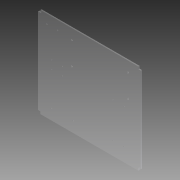
# Autodesk Inventor part: base plate
Saved by Autodesk Inventor 2012 (Build 160160000, 160)
## iProperties
Created: 2012-03-15
Part Number: base plate
Material: Polycarbonate, Clear
Document SubType Name: Modeling
Designer: Ed
Mass: 1928.1 g
Surface Area: 5188.7 cm^2
Volume: 1606.75 cm^3
Density: 1.2 g/cm^3
Author: Ed
Autodesk Inventor part; units mm, degrees
ref_plane "YZ Plane" through (0, 0, 0) normal (1, 0, 0) x (0, 1, 0)
ref_plane "XZ Plane" through (0, 0, 0) normal (0, 1, 0) x (-1, 0, 0)
ref_plane "XY Plane" through (0, 0, 0) normal (0, 0, 1) x (1, 0, 0)
sketch "Sketch1" plane through (0, 0, 0) normal (0, 0, 1) x (1, 0, 0)
  line L0 (0, 0) -> (546.1, 0)
  line L1 (546.1, 0) -> (546.1, 479.425)
  line L2 (546.1, 479.425) -> (0, 479.425)
  line L3 (0, 479.425) -> (0, 0)
  line L4 (0, 0) -> (12.7, 0)
  line L5 (12.7, 0) -> (12.7, 12.7)
  line L6 (12.7, 12.7) -> (0, 12.7)
  line L7 (0, 12.7) -> (0, 0)
  line L8 (0, 479.425) -> (12.7, 479.425)
  line L9 (12.7, 479.425) -> (12.7, 466.725)
  line L10 (12.7, 466.725) -> (0, 466.725)
  line L11 (0, 466.725) -> (0, 479.425)
  line L12 (546.1, 479.425) -> (533.4, 479.425)
  line L13 (533.4, 479.425) -> (533.4, 466.725)
  line L14 (533.4, 466.725) -> (546.1, 466.725)
  line L15 (546.1, 466.725) -> (546.1, 479.425)
  line L16 (546.1, 0) -> (533.4, 0)
  line L17 (533.4, 0) -> (533.4, 12.7)
  line L18 (533.4, 12.7) -> (546.1, 12.7)
  line L19 (546.1, 12.7) -> (546.1, 0)
  dimension "d0" = 479.425
  dimension "d1" = 546.1
  dimension "d2" = 12.7
  constraints: 40 end point, 10 parallel, 7 equal length, 5 horizontal, 5 perpendicular
  measures "d0" distance of L2.end L0.start
  measures "d1" distance of L0.start L0.end
  measures "d2" distance of L8.end L9.end
extrude "Lexan Plate" add sketch "Sketch1" along normal blind 6.35 contours L5 L6 L3 L10 L9 L2 L13 L14 L1 L18 L17 L0
sketch "Sketch2" plane through (0, 0, 6.35) normal (0, 0, 1) x (1, 0, 0)
  line L0 (12.7, 479.425) -> (533.4, 479.425) projected
  line L1 (546.1, 466.725) -> (546.1, 12.7) projected
  line L2 (476.25, 301.625) -> (177.8, 301.625)
  line L3 (177.8, 301.625) -> (177.8, 422.275)
  line L4 (177.8, 422.275) -> (476.25, 422.275)
  line L5 (476.25, 422.275) -> (476.25, 301.625)
  point P0 (0, 0)
  dimension "d7" = 69.85
  dimension "d8" = 57.15
  dimension "d9" = 120.65
  dimension "d10" = 298.45
  constraints: 8 end point, 4 coincident, 2 parallel, 1 horizontal, 1 perpendicular
  measures "d7" distance between parallel lines of L1 L5
  measures "d8" distance between parallel lines of L4 L0
  measures "d9" distance of L4.end L2.start
  measures "d10" distance of L3.end L4.end
hole "Inverter Mounting Holes" at (177.8, 422.275, 6.35) at (177.8, 301.625, 6.35) at (476.25, 301.625, 6.35) at (476.25, 422.275, 6.35) direction (0, 0, -1) diameter 6.7564 end through all clearance for "Flat Head Machine Screw (82)" size "1/4" standard "Ansi Unified Screw Threads"
sketch "Sketch3" plane through (0, 0, 6.35) normal (0, 0, 1) x (1, 0, 0)
  line L0 (533.4, 0) -> (12.7, 0) projected
  line L1 (546.1, 466.725) -> (546.1, 12.7) projected
  line L2 (394.4938, 255.5875) -> (454.025, 255.5875)
  line L3 (454.025, 255.5875) -> (454.025, 69.85)
  line L4 (454.025, 69.85) -> (394.4938, 69.85)
  line L5 (394.4938, 69.85) -> (394.4938, 255.5875)
  point P0 (0, 0)
  dimension "d18" = 69.85
  dimension "d19" = 92.075
  dimension "d20" = 59.5312
  dimension "d21" = 185.7375
  constraints: 8 end point, 4 coincident, 2 parallel, 1 horizontal, 1 perpendicular
  measures "d18" distance between parallel lines of L0 L4
  measures "d19" distance between parallel lines of L1 L3
  measures "d20" distance of L3.end L4.end
  measures "d21" distance of L2.end L3.end
hole "13.8v Supply Mounting Holes" at (394.4938, 255.5875, 6.35) at (454.025, 255.5875, 6.35) at (454.025, 69.85, 6.35) at (394.4938, 69.85, 6.35) direction (0, 0, -1) diameter 3.9624 end through all thread size "10-32 UNF" class "2B" standard "ANSI Unified Screw Threads"
sketch "Sketch4" plane through (0, 0, 6.35) normal (0, 0, 1) x (1, 0, 0)
  line L0 (0, 12.7) -> (0, 466.725) projected
  line L1 (533.4, 0) -> (12.7, 0) projected
  line L2 (546.1, 466.725) -> (533.4, 466.725) projected
  line L3 (69.85, 53.975) -> (184.15, 53.975)
  point P0 (0, 0)
  dimension "d29" = 69.85
  dimension "d30" = 114.3
  dimension "d31" = 53.975
  constraints: 2 coincident, 2 end point, 1 parallel
  measures "d29" distance from line of L0 L3.start
  measures "d30" distance of L3.start L3.end
  measures "d31" distance between parallel lines of L1 L3
hole "cRIO Mounting Holes" at (184.15, 53.975, 6.35) at (69.85, 53.975, 6.35) direction (0, 0, -1) diameter 3.9624 end through all thread size "10-32 UNF" class "2B" standard "ANSI Unified Screw Threads"
sketch "Sketch5" plane through (0, 0, 6.35) normal (0, 0, 1) x (1, 0, 0)
  line L0 (0, 12.7) -> (0, 466.725) projected
  line L1 (533.4, 0) -> (12.7, 0) projected
  line L2 (69.85, 276.225) -> (127, 276.225)
  line L3 (127, 276.225) -> (127, 231.775)
  line L4 (127, 231.775) -> (69.85, 231.775)
  line L5 (69.85, 231.775) -> (69.85, 276.225)
  point P0 (0, 0)
  dimension "d40" = 44.45
  dimension "d41" = 57.15
  dimension "d42" = 69.85
  dimension "d43" = 231.775
  constraints: 8 end point, 4 coincident, 2 parallel, 1 horizontal, 1 perpendicular
  measures "d40" distance of L4.end L2.start
  measures "d41" distance of L3.end L4.end
  measures "d42" distance between parallel lines of L0 L5
  measures "d43" distance between parallel lines of L1 L4
hole "Sabertooth Mounting Holes" at (127, 276.225, 6.35) at (127, 231.775, 6.35) at (69.85, 231.775, 6.35) at (69.85, 276.225, 6.35) direction (0, 0, -1) diameter 2.159 end through all
sketch "Sketch6" plane through (0, 0, 6.35) normal (0, 0, 1) x (1, 0, 0)
  line L0 (12.7, 479.425) -> (533.4, 479.425) projected
  line L1 (0, 12.7) -> (0, 466.725) projected
  line L2 (546.1, 466.725) -> (533.4, 466.725) projected
  line L3 (44.45, 428.625) -> (101.6, 428.625)
  point P0 (0, 0)
  dimension "d51" = 57.15
  dimension "d52" = 44.45
  dimension "d53" = 50.8
  constraints: 2 coincident, 2 end point, 1 parallel
  measures "d51" distance of L3.start L3.end
  measures "d52" distance from line of L3.start L1
  measures "d53" distance between parallel lines of L0 L3
hole "Estop Relay Mounting Holes" at (101.6, 428.625, 6.35) at (44.45, 428.625, 6.35) direction (0, 0, -1) diameter 4.9784 end through all thread size "1/4-20 UNC" class "2B" standard "ANSI Unified Screw Threads"
body "Solid2"
